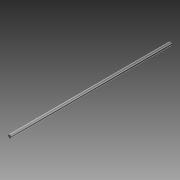
# Autodesk Inventor part: m8_rail
Saved by Autodesk Inventor 2014 SP2 (Build 180246200, 246)
## iProperties
Created: 2014-07-14
Part Number: m8_rail
Material: Generic
Document SubType Name: Modeling
Designer: cruiser
Density: 1 g/cm^3
Appearance: Stainless Steel - Bright
Author: cruiser
Autodesk Inventor part; units mm, degrees
ref_plane "YZ Plane" through (0, 0, 0) normal (1, 0, 0) x (0, 1, 0)
ref_plane "XZ Plane" through (0, 0, 0) normal (0, 1, 0) x (-1, 0, 0)
ref_plane "XY Plane" through (0, 0, 0) normal (0, 0, 1) x (1, 0, 0)
sketch "Sketch1" plane through (0, 0, 0) normal (0, 1, 0) x (-1, 0, 0)
  circle A0 centre (0, 0) radius 4
  dimension "d0" = 8
  constraints: 1 centre point, 1 coincident
  measures "d0" diameter of A0
extrude "Extrusion1" add sketch "Sketch1" along normal blind 400
equation "\"d1\" = m8_rail_height"
equation "\"m8_rail_height\" = linear_bearing_z"
equation "\"sm_thickness\" = 1.5875"
equation "\"very_thick_acrylic\" = 9.45"
equation "\"thick_acrylic\" = 5.88"
equation "\"thin_acrylic\" = 3.15"
equation "\"clear_acrylic\" = 3.15"
equation "\"wood_thickness\" = 6.72"
equation "\"m3_diameter\" = 3"
equation "\"m3_head\" = 6"
equation "\"m4_diameter\" = 4"
equation "\"m5_diameter\" = 5"
equation "\"brass_insert_drill\" = 4"
equation "\"m5_brass_insert_drill\" = 6.7"
equation "\"m3_press_nut_drill\" = 4.5"
equation "\"m3_main_length\" = 14"
equation "\"m3_main_nut_width\" = 5.7"
equation "\"m3_main_nut_thickness\" = 2.5"
equation "\"m3_main_extra\" = 1"
equation "\"stepper_screw_space\" = 35"
equation "\"stepper_shaft_diameter\" = 5"
equation "\"stepper_body_diameter\" = 28"
equation "\"laser_body_diameter\" = 12"
equation "\"carrier_y\" = 251"
equation "\"carrier_z\" = 12"
equation "\"visor_x\" = 257.3"
equation "\"visor_y\" = 110.2375"
equation "\"window_z\" = 333.9125"
equation "\"window_y\" = 92.0625"
equation "\"window_overlap\" = 48"
equation "\"acrylic_into_frame\" = 5"
equation "\"door_x\" = 251"
equation "\"door_z\" = 333.9125"
equation "\"door_overlap\" = 48"
equation "\"reservoir_x\" = 201"
equation "\"reservoir_y\" = 201"
equation "\"linear_bearing_spacing\" = 271"
equation "\"motor_spacing\" = 337"
equation "\"tray_border\" = 25"
equation "\"tray_x\" = 251"
equation "\"tray_y\" = 251"
equation "\"bed_z\" = 25"
equation "\"crane_z2\" = 12"
equation "\"end_stop_spacing\" = 19"
equation "\"thumb_nut_offset_y\" = 0"
equation "\"thumb_nut_diameter\" = 7"
equation "\"z_min_from_center\" = 115"
equation "\"frame_top_z\" = 385"
equation "\"frame_bottom_z\" = 275"
equation "\"frame_total_z\" = 661.5875"
equation "\"frame_border\" = 46.35"
equation "\"frame_foot_z\" = 12"
equation "\"frame_tilt\" = 1deg"
equation "\"printer_z\" = 289"
equation "\"lcd_x\" = 72"
equation "\"lcd_y\" = 25"
equation "\"subframe_x\" = 195"
equation "\"subframe_y_offset\" = 27.5"
equation "\"laser_y_offset\" = 19.4"
equation "\"laser_diameter\" = 12"
equation "\"laser_z_offset\" = 55"
equation "\"laser_y\" = 15"
equation "\"laser_z\" = 75"
equation "\"t_galvo_frame\" = 6.72"
equation "\"galvo_frame_x\" = 66"
equation "\"galvo_frame_z\" = 65"
equation "\"galvo_frame_y_offset\" = 27.5"
equation "\"drawer_x\" = 257.3"
equation "\"drawer_y\" = 88.65"
equation "\"drawer_z\" = 278.175"
equation "\"drawer_z_from_bottom\" = 25"
equation "\"nema17_x\" = 43"
equation "\"m5_press_nut_drill\" = 6.5"
equation "\"drawer_support_from_top\" = 48"
equation "\"laser_gap\" = 1"
equation "\"frame_screw_from_center\" = 25"
equation "\"magnet_z\" = 45"
equation "\"drawer_screw_z\" = 117"
equation "\"frame_face_y\" = 44"
equation "\"switch_spacing\" = 19"
equation "\"linear_bearing_z\" = 400"
body "Solid1"
